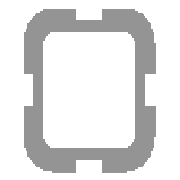
# Autodesk Inventor part: CE-5.2.2-PR
Saved by Autodesk Inventor 2024 (Build 280153000, 153)
## iProperties
Created: 2024-02-15
Part Number: CE-5.2.2-PR
Material: Generic
Document SubType Name: Modeling
Designer: Alex
Density: 1 g/cm^3
Appearance: Default
Categories: <MemberInstance><Categories><Category DisplayName="Structural Shapes" InternalName="089c4875-fa83-4c05-b084-43b9cc11f5ed" Mnemonic="GRDR"><CategoryParameter DisplayName="Mass per Length Unit" InternalName="0bb95a10-148f-4027-a459-38d7b056702a" Mnemonic="shpmass"/><CategoryParameter DisplayName="Section Area" InternalName="1ff91680-64b0-4202-b9a3-7fd3f94bba3b" Mnemonic="secarea"/><CategoryParameter DisplayName="Radius of Gyration (x)" InternalName="25778675-03e9-40c1-b6a8-4a9ed693320d" Mnemonic="gyrradx"/><CategoryParameter DisplayName="Torsional Rigidity Modulus" InternalName="26c1ec35-5026-4c63-ad0a-751cf684a536" Mnemonic="torrigmod"/><CategoryParameter DisplayName="Distance of the Center of Gravity X-X" InternalName="26c9bdb8-9c79-4b4f-a92e-8e197583c9c4" Mnemonic="grcendistX"/><CategoryParameter DisplayName="Legacy Member ID" InternalName="340afe4f-75d7-48d3-ab7d-943f3c3da468" Mnemonic="LegacyMemberID"/><CategoryParameter DisplayName="Base Length" InternalName="42e34263-8f20-4d0e-ad48-bf1385b87c24" Mnemonic="shplen"/><CategoryParameter DisplayName="Moment of Inertia (y)" InternalName="4b9f58ea-bced-460e-81ea-3d29ca5a49e3" Mnemonic="inermomy"/><CategoryParameter DisplayName="Moment of Inertia (x)" InternalName="4cd780bc-73d7-43ac-917a-579e5cbd684d" Mnemonic="inermomx"/><CategoryParameter DisplayName="Custom Base Point" InternalName="4f1d1b73-316d-484b-a3df-9cbabb16eb77" Mnemonic="shpBasePoint"/><CategoryParameter DisplayName="Shape Height" InternalName="50274e7d-5ac0-4796-92cb-c59e54983c67" Mnemonic="shpheig"/><CategoryParameter DisplayName="Section Module (y)" InternalName="59eaa5e9-d227-48dc-b6c1-6920f96e0f95" Mnemonic="secmody"/><CategoryParameter DisplayName="Section Designation" InternalName="5a64d034-428d-49c8-ba32-7619764de20f" Mnemonic="shpdes"/><CategoryParameter DisplayName="Section Module (x)" InternalName="72cfad18-cf51-4ed4-aaa7-c6b224f8419f" Mnemonic="secmodx"/><CategoryParameter DisplayName="Torsional Section Modulus" InternalName="7c55a8dc-8844-49f9-a867-cc677b30ec9a" Mnemonic="torsecmod"/><CategoryParameter DisplayName="Shape Width" InternalName="7c717d54-a18f-4666-b4d4-573cce22c62c" Mnemonic="shpwdth"/><CategoryParameter DisplayName="Second Shape Thickness" InternalName="9251a8e1-85fd-4e47-af99-afdb762317d9" Mnemonic="shpthick2"/><CategoryParameter DisplayName="FG Authored" InternalName="9c666724-f362-4ea7-ac62-f6a007de5c69" Mnemonic="shpFGAuto"/><CategoryParameter DisplayName="Distance of the Center of Gravity Y-Y" InternalName="bcc4fb17-7af4-436a-8f8c-d0aa3b0248c5" Mnemonic="grcendistY"/><CategoryParameter DisplayName="Radius of Gyration (y)" InternalName="bfa18ebe-1636-4dbe-8d42-b263e0b73184" Mnemonic="gyrrady"/><CategoryParameter DisplayName="Shape Thickness" InternalName="d109cf76-8eb4-42fc-9800-4409734adc67" Mnemonic="shpthick"/><CategoryParameter DisplayName="Coefficient of Shear Displacement" InternalName="de4c90c6-aaa8-468f-a335-6737b311b5d3" Mnemonic="shdispc"/><Category DisplayName="Square/Rectangular Tubes" InternalName="afc8e2d8-05d6-4609-8807-f98a9b7d2ed0" Mnemonic="SQRSHP"><CategoryParameter DisplayName="Section Area" InternalName="2f7f79dd-983c-4263-802a-5b6a1495fdc5" Mnemonic="secarea"/><CategoryParameter DisplayName="Section Module (x)" InternalName="50d965a6-04bf-46b9-8ace-861858d348e6" Mnemonic="secmodx"/><CategoryParameter DisplayName="Section Module (y)" InternalName="5106aeac-54a2-4159-a9af-8933dd39dba2" Mnemonic="secmody"/><CategoryParameter DisplayName="Shape Thickness" InternalName="52712fc5-f4ee-4eda-b3f2-6fce82c26419" Mnemonic="shpthick"/><CategoryParameter DisplayName="Moment of Inertia (y)" InternalName="55ec8510-8276-4c45-8f10-594e0fee7eb3" Mnemonic="inermomy"/><CategoryParameter DisplayName="Radius of Gyration (x)" InternalName="56c89926-a299-4389-a862-ac94c9691272" Mnemonic="gyrradx"/><CategoryParameter DisplayName="Radius" InternalName="5d8d062c-e28e-41c1-98da-8e5fee36da1a" Mnemonic="shprad"/><CategoryParameter DisplayName="Moment of Inertia (x)" InternalName="8c4637b6-6b69-4878-9d5d-26a32185d655" Mnemonic="inermomx"/><CategoryParameter DisplayName="Shape Width" InternalName="8c8a1782-5e80-4d77-858b-304b1c0ad1fd" Mnemonic="shpwdth"/><CategoryParameter DisplayName="Radius of Gyration (y)" InternalName="fa48a7f5-f030-40f9-a60b-de8a845b7104" Mnemonic="gyrrady"/></Category></Category></Categories><FamilyTemplate Id="CE-5.2.2-PR"><FamilyTemplateParameters><FamilyTemplateParameter ObjectType="kModelParameterObject" ValueType="xs:double" Id="12" ObjectReferenceKey="Length"/></FamilyTemplateParameters></FamilyTemplate><CategoryParameterMap><ParamToTemplateMap><ParamToTemplate CategoryParameter="//CategoryParameter[@InternalName='42e34263-8f20-4d0e-ad48-bf1385b87c24']" TemplateParameter="12"/><ParamToTemplate CategoryParameter="//CategoryParameter[@InternalName='9c666724-f362-4ea7-ac62-f6a007de5c69']" ConstantValue="1"/></ParamToTemplateMap></CategoryParameterMap></MemberInstance>
G_L: 50.000 mm
Author: Alex
Autodesk Inventor part; units mm, degrees
ref_plane "YZ Plane" through (0, 0, 0) normal (1, 0, 0) x (0, 1, 0)
ref_plane "Start Plane" through (0, 0, 0) normal (0, 1, 0) x (-1, 0, 0)
ref_plane "End Plane" through (0, 50, 0) normal (0, 1, 0) x (-1, 0, 0)
sketch "Sketch1" plane through (0, 0, 0) normal (0, 1, 0) x (-1, 0, 0)
  line L0 (8, -10) -> (-8, -10)
  line L1 (-10, -8) -> (-10, 8)
  line L2 (-8, 10) -> (8, 10)
  line L3 (10, 8) -> (10, -8)
  line L4 (10, -10) -> (-10, 10) construction
  line L5 (-10, -10) -> (10, 10) construction
  line L6 (14, -14) -> (-14, 14) construction
  line L7 (-14, -14) -> (14, 14) construction
  arc A0 (8, -10) -> (10, -8) centre (8, -8) ccw
  arc A1 (-10, -8) -> (-8, -10) centre (-8, -8) ccw
  arc A2 (-8, 10) -> (-10, 8) centre (-8, 8) ccw
  arc A3 (10, 8) -> (8, 10) centre (8, 8) ccw
  arc A4 (8, -14) -> (14, -8) centre (8, -8) ccw
  arc A5 (-14, -8) -> (-8, -14) centre (-8, -8) ccw
  arc A6 (-8, 14) -> (-14, 8) centre (-8, 8) ccw
  arc A7 (14, 8) -> (8, 14) centre (8, 8) ccw
  line L8 (3, -14) -> (3, -12)
  line L9 (3, -12) -> (-3, -12)
  line L10 (-3, -12) -> (-3, -14)
  line L11 (-14, -3) -> (-12, -3)
  line L12 (-12, -3) -> (-12, 3)
  line L13 (-12, 3) -> (-14, 3)
  line L14 (-3, 14) -> (-3, 12)
  line L15 (-3, 12) -> (3, 12)
  line L16 (3, 12) -> (3, 14)
  line L17 (14, 3) -> (12, 3)
  line L18 (12, 3) -> (12, -3)
  line L19 (12, -3) -> (14, -3)
  line L20 (0, -10) -> (0, -12) construction
  line L21 (-10, 0) -> (-12, 0) construction
  line L22 (0, 10) -> (0, 12) construction
  line L23 (10, 0) -> (12, 0) construction
  line L24 (14, 8) -> (14, 3)
  line L25 (14, -3) -> (14, -8)
  line L26 (8, -14) -> (3, -14)
  line L27 (-3, -14) -> (-8, -14)
  line L28 (-14, -8) -> (-14, -3)
  line L29 (-14, 3) -> (-14, 8)
  line L30 (-8, 14) -> (-3, 14)
  line L31 (3, 14) -> (8, 14)
  point P0 (0, 0)
  dimension "d1" = 20
  dimension "d2" = 2
  dimension "d3" = 6
  dimension "d4" = 20
  dimension "d5" = 6
  dimension "d6" = 2
  dimension "d8" = 28
  constraints: 64 end point, 33 perpendicular, 24 tangent, 16 point on circle, 12 midpoint, 10 parallel, 9 point on line, 8 centre point, 6 equal radius, 5 horizontal, 3 vertical
  measures "d1" distance of L4.start L5.start
  measures "d2" radius of A0
  measures "d3" radius of A4
  measures "d4" distance between parallel lines of L2 L0
  measures "d5" distance of L8.end L9.end
  measures "d6" distance of L11.start L11.end
  measures "d8" distance between parallel lines of L28 L25
extrude "Body" add sketch "Sketch1" along normal up to surface (50 mm away) from surface at 0
sketch "Sketch2" plane through (0, 0, 0) normal (0, 1, 0) x (-1, 0, 0)
  line L0 (0, 0) -> (10, 0)
ref_plane "Work Plane3" through (0, 0, 0) normal (0, 0, -1) x (-1, 0, 0)
sketch "Sketch3" plane through (0, 0, 0) normal (0, 0, -1) x (-1, 0, 0)
  line L0 (-19.6, 0) -> (19.6, 0) construction
  line L1 (-19.6, 50) -> (19.6, 50) construction
  dimension "d16" = 50
  measures "d16" distance between parallel lines of L0 L1
equation "\"G_OFFSET_START\" = 0"
equation "\"G_OFFSET_END\" = 0"
equation "\"G_L\" = d16"
body "Solid1"
